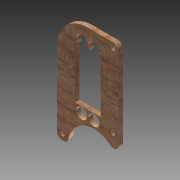
# Autodesk Inventor part: p1
Saved by Autodesk Inventor 2015 (Build 190159000, 159)
## iProperties
Created: 2016-02-03
Part Number: p1
Material: Generic
Document SubType Name: Modeling
Designer: david
Density: 1 g/cm^3
Appearance: Birch - Natural Polished
Mass: 8.91381 g
Surface Area: 67.6659 cm^2
Volume: 8.91381 cm^3
Author: david
Autodesk Inventor part; units mm, degrees
ref_plane "YZ Plane" through (0, 0, 0) normal (1, 0, 0) x (0, 1, 0)
ref_plane "XZ Plane" through (0, 0, 0) normal (0, 1, 0) x (-1, 0, 0)
ref_plane "XY Plane" through (0, 0, 0) normal (0, 0, 1) x (1, 0, 0)
sketch "Sketch1" plane through (0, 0, 0) normal (0, 1, 0) x (-1, 0, 0)
  line L0 (20, 45) -> (-20, 45)
  line L1 (-20, 45) -> (-20, -45)
  line L2 (-20, -45) -> (20, -45)
  line L3 (20, -45) -> (20, 45)
  line L4 (20, 45) -> (-20, -45) construction
  line L5 (-20, 45) -> (20, -45) construction
  arc A0 (-20, -45) -> (20, -45) centre (0, -45) ccw
  line L6 (20, -45) -> (30, -45)
  line L7 (30, -45) -> (30, 45)
  line L8 (30, 45) -> (20, 45)
  line L9 (20, 45) -> (20, -45)
  point P0 (0, 0)
  dimension "d0" = 40
  dimension "d1" = 90
  dimension "d7" = 10
  dimension "d8" = 90
  constraints: 20 end point, 4 parallel, 3 midpoint, 2 horizontal, 2 perpendicular, 2 point on circle, 1 centre point
  measures "d0" distance of L2.end L1.end
  measures "d1" distance of L1.end L0.end
  measures "d7" distance of L8.end L7.end
  measures "d8" distance of L7.end L6.end
extrude "Extrusion1" add sketch "Sketch1" along normal blind 3.6
fillet "Fillet1" radius 4 3 edges at (-20, 1.8, -45) (-30, 1.8, -45) (20, 1.8, 45)
sketch "Sketch3" plane through (0, 0, 0) normal (0, -1, 0) x (1, 0, 0)
  circle A0 centre (0, -45) radius 21
  arc A1 (-19.7203, -48.3333) -> (20, -45) centre (0, -45) ccw projected
  point P0 (0, 0)
  dimension "d10" = 42
  dimension "d11" = 0
  constraints: 1 centre point
  measures "d10" diameter of A0
  measures "d11" distance of A1.centre A0.centre
extrude "Extrusion3" cut sketch "Sketch3" against normal blind 10
fillet "Fillet2" radius 4 2 edges at (20, 1.8, -38.5969) (-20.9742, 1.8, -46.0397)
sketch "Sketch4" plane through (0, 0, 0) normal (0, -1, 0) x (1, 0, 0)
  circle A0 centre (-25.5, -40.5) radius 1.625
  line L0 (-24.6779, -45) -> (-26, -45) projected
  circle A1 centre (15.5, -19.5) radius 1.625
  circle A2 centre (15.5, 40.5) radius 1.625
  line L1 (20, 41) -> (20, -25.7906) projected
  arc A3 (13.44, -28.8641) -> (20, -25.7906) centre (16, -25.7906) ccw projected
  line L2 (-30, -41) -> (-30, 45) projected
  line L3 (-30, 45) -> (16, 45) projected
  point P0 (0, 0)
  point P1 (-30, 41)
  point P2 (-26, 45)
  dimension "d15" = 3.25
  dimension "d16" = 4.5
  dimension "d21" = 3.25
  dimension "d22" = 3.25
  dimension "d23" = 4.5
  dimension "d25" = 4.5
  dimension "d29" = 4.5
  dimension "d30" = 4.5
  dimension "d31" = 60
  constraints: 3 centre point
  measures "d15" diameter of A0
  measures "d16" distance from line of L0 A0.centre
  measures "d21" diameter of A1
  measures "d22" diameter of A2
  measures "d23" distance from line of L1 A1.centre
  measures "d25" distance from line of L1 A2.centre
  measures "d29" distance from line of L2 A0.centre
  measures "d30" distance from line of A2.centre L3
  measures "d31" distance of A2.centre A1.centre
extrude "Extrusion4" cut sketch "Sketch4" against normal blind 7
sketch "Sketch5" plane through (0, 0, 0) normal (0, -1, 0) x (1, 0, 0)
  line L0 (-15.5, 30) -> (5.5, 30)
  line L1 (5.5, 30) -> (5.5, -13)
  line L2 (5.5, -13) -> (-15.5, -13)
  line L3 (-15.5, -13) -> (-15.5, 30)
  line L4 (-15.5, 30) -> (5.5, -13) construction
  line L5 (5.5, 30) -> (-15.5, -13) construction
  line L6 (-24.6779, -45) -> (-26, -45) projected
  line L7 (-30, -41) -> (-30, 45) projected
  point P0 (0, 0)
  point P1 (-5, 8.5)
  point P2 (-30, 41)
  dimension "d32" = 21
  dimension "d33" = 43
  dimension "d34" = 32
  dimension "d35" = 14.5
  constraints: 12 end point, 2 midpoint, 2 parallel, 1 horizontal, 1 perpendicular
  measures "d32" distance of L1.end L2.end
  measures "d33" distance of L0.end L1.end
  measures "d34" distance between parallel lines of L6 L2
  measures "d35" distance between parallel lines of L7 L3
extrude "Extrusion5" cut sketch "Sketch5" against normal blind 10
sketch "Sketch6" plane through (0, 0, 0) normal (0, -1, 0) x (1, 0, 0)
  circle A0 centre (0, -18) radius 4.5
  circle A1 centre (0, 33) radius 4.5
  circle A2 centre (-10, -18) radius 4.5
  circle A3 centre (-10, 33) radius 4.5
  line L0 (5.5, 30) -> (5.5, -13) projected
  line L1 (5.5, -13) -> (-15.5, -13) projected
  point P0 (0, 0)
  dimension "d38" = 9
  dimension "d39" = 9
  dimension "d40" = 51
  dimension "d41" = 9
  dimension "d42" = 9
  dimension "d43" = 10
  dimension "d44" = 10
  dimension "d45" = 51
  dimension "d46" = 90
  dimension "d47" = 5.5
  dimension "d48" = 5
  constraints: 4 centre point
  measures "d38" diameter of A0
  measures "d39" diameter of A1
  measures "d40" distance of A1.centre A0.centre
  measures "d41" diameter of A2
  measures "d42" diameter of A3
  measures "d43" distance of A2.centre A0.centre
  measures "d44" distance of A3.centre A1.centre
  measures "d45" distance of A2.centre A3.centre
  measures "d47" distance from line of L0 A0.centre
  measures "d48" distance from line of L1 A0.centre
extrude "Extrusion6" cut sketch "Sketch6" against normal blind 10
fillet "Fillet3" radius 25 1 edges at (-30, 1.8, 45)
body "Solid1"
